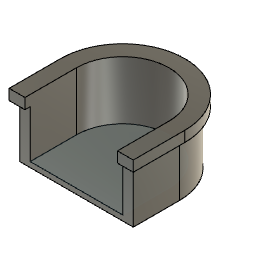
turnknob holder v5 (Autodesk Fusion 360 design; units mm, degrees)
Autodesk Fusion 360 part; units mm, degrees
note: some values were not read from the file. Chosen so that the rebuilt part matches the saved one: which face or edge a step refers to. Set by a fixed rule: which sketch regions a step uses.
sketch "Sketch1" plane through (0, 0, 0) normal (0, 0, 1) x (1, 0, 0)
  line L0 (-8.75, 0) -> (-8.75, -8.75)
  line L1 (-8.75, -8.75) -> (0, -8.75)
  line L2 (0, -8.75) -> (8.75, -8.75)
  line L3 (8.75, -8.75) -> (8.75, 0)
  arc A0 (8.75, 0) -> (-8.75, 0) centre (0, 0) ccw
  line L4 (10.75, -8.75) -> (10.75, 0)
  arc A1 (10.75, 0) -> (-10.75, 0) centre (0, 0) ccw
  line L5 (-10.75, 0) -> (-10.75, -8.75)
  line L6 (-8.75, -8.75) -> (-10.75, -8.75)
  line L7 (8.75, -8.75) -> (10.75, -8.75)
  dimension "d8" = 17.5
  dimension "d9" = 8.75
  dimension "d10" = 8.75
  dimension "d25" = 2
  constraint coincident A0.centre A1.centre
  constraint tangent L0 A0
  constraint tangent L1 A0
  constraint tangent L2 A0
  constraint tangent L3 A0
  constraint perpendicular L5 L6
  constraint perpendicular L4 L7
  constraint parallel L3 L4
  constraint concentric A0 A1
  constraint parallel L0 L5
  constraint tangent A1 L5
  constraint tangent L4 A1
  measures "d8" diameter of A0
  measures "d9" distance of L0.start L0.end
  measures "d10" distance of L1.end L2.end
  measures "d25" distance of L0.end L5.end
extrude "Extrude4" add sketch "Sketch1" along normal blind 1
sketch "Sketch4" plane through (0, 0, 1) normal (0, 0, 1) x (-1, 0, 0)
  line L0 (10.75, 8.75) -> (-10.75, 8.75)
  line L1 (-8.75, 7.75) -> (-8.75, 0)
  arc A0 (-8.75, 0) -> (8.75, 0) centre (0, 0) ccw
  line L2 (8.75, 0) -> (8.75, 7.75)
  line L3 (8.75, 7.75) -> (8.75, 8.75)
  line L4 (-8.75, 7.75) -> (-8.75, 8.75)
  line L5 (-8.75, 8.75) -> (8.75, 8.75)
  line L6 (-10.75, 8.75) -> (-10.75, 0)
  arc A1 (-10.75, 0) -> (10.75, 0) centre (0, 0) ccw
  line L7 (10.75, 0) -> (10.75, 8.75)
  constraint coincident L0 L3.end
  constraint perpendicular L0 L3
  constraint coincident L0 L4.end
  constraint perpendicular L0 L4
  constraint tangent L1 A0
  constraint tangent A0 L2
extrude "Extrude5" add sketch "Sketch4" along normal blind 10.5 contours L0 L1 A0 L2 L3 L4 L6 A1 L7
extrude "Extrude7" add 1 faces at (10.0833, -5.8333, 11.5) along direction (0, 0, 1) blind 0.5
sketch "Sketch7" plane through (0, 0, 12) normal (0, 0, 1) x (-1, 0, 0)
  line L0 (-10.75, 8.75) -> (-10.75, 0)
  arc A0 (-10.75, 0) -> (10.75, 0) centre (0, 0) ccw
  line L1 (10.75, 0) -> (10.75, 8.75)
  line L2 (10.75, 8.75) -> (8.75, 8.75)
  line L3 (8.75, 8.75) -> (8.75, 0)
  arc A1 (-8.75, 0) -> (8.75, 0) centre (0, 0) ccw
  line L4 (-8.75, 0) -> (-8.75, 8.75)
  line L5 (-8.75, 8.75) -> (-10.75, 8.75)
  arc A2 (-11.75, 0) -> (11.75, 0) centre (0, 0) ccw
  line L6 (11.75, 0) -> (11.75, 9.75)
  line L7 (11.75, 9.75) -> (7.75, 9.75)
  line L8 (7.75, 9.75) -> (7.75, 0)
  arc A3 (-7.75, 0) -> (7.75, 0) centre (0, 0) ccw
  line L9 (-7.75, 0) -> (-7.75, 9.75)
  line L10 (-7.75, 9.75) -> (-11.75, 9.75)
  line L11 (-11.75, 9.75) -> (-11.75, 0)
  dimension "d28" = 1
extrude "Extrude8" add sketch "Sketch7" against normal blind 2
sketch "Sketch8" plane through (0, 0, 12) normal (0, 0, 1) x (-1, 0, 0)
  line L0 (-7.75, 0) -> (-7.75, 9.75)
  line L1 (-7.75, 9.75) -> (-11.75, 9.75)
  line L2 (-11.75, 9.75) -> (-11.75, 0)
  arc A0 (-11.75, 0) -> (11.75, 0) centre (0, 0) ccw
  line L3 (11.75, 0) -> (11.75, 9.75)
  line L4 (11.75, 9.75) -> (7.75, 9.75)
  line L5 (7.75, 9.75) -> (7.75, 0)
  arc A1 (-7.75, 0) -> (7.75, 0) centre (0, 0) ccw
  circle A2 centre (0, 0) radius 8.75
  line L6 (8.75, 9.75) -> (7.75, 9.75)
  line L7 (7.75, 9.75) -> (-7.75, 9.75)
  line L8 (-7.75, 9.75) -> (-8.75, 9.75)
  line L9 (-8.75, 9.75) -> (-8.75, 0)
  line L10 (8.75, 9.75) -> (8.75, 0)
  dimension "d31" = 17.5
  dimension "d32" = 1
  constraint concentric A0 A2
  constraint coincident A2 L10.end
  constraint coincident L4 L6.start
  constraint coincident L4.end L5.start
  constraint perpendicular L5 L6
  constraint coincident L0.end L1.start
  constraint coincident L1 L8.end
  constraint coincident A2 L9.end
  constraint tangent A2 L9
  constraint tangent A2 L10
  measures "d31" diameter of A2
  measures "d32" distance of L0.end L8.end
extrude "Extrude9" cut sketch "Sketch8" against normal blind 11 contours L0 L5 A1 A2 | L0 L5 A1 A2 | L0 L1 A2 L8 L9 | L4 L5 A2 L6 L10
sketch "Sketch9" plane through (0, 0, 1) normal (0, 0, 1) x (-1, 0, 0)
  line L0 (8.75, 8.75) -> (-8.75, 8.75)
  line L1 (-8.75, 8.75) -> (-8.75, 0)
  arc A0 (-8.75, 0) -> (8.75, 0) centre (0, 0) ccw
  line L2 (8.75, 0) -> (8.75, 8.75)
sketch "Sketch5" plane through (0, 0, 9.5) normal (0, 0, 1) x (-1, 0, 0)
  line L0 (-8.75, 0) -> (-8.75, 8.75)
  line L1 (-8.75, 8.75) -> (-9.75, 8.75)
  line L2 (-9.75, 8.75) -> (-9.75, 0)
  arc A0 (-9.75, 0) -> (9.75, 0) centre (0, 0) ccw
  line L3 (9.75, 0) -> (9.75, 8.75)
  line L4 (9.75, 8.75) -> (8.75, 8.75)
  line L5 (8.75, 8.75) -> (8.75, 0)
  arc A1 (-8.75, 0) -> (8.75, 0) centre (0, 0) ccw
  arc A2 (-10.75, 0) -> (10.75, 0) centre (0, 0) ccw
  line L6 (-10.75, 0) -> (-10.75, 8.75)
  line L7 (-10.75, 8.75) -> (-9.75, 8.75)
  line L8 (10.75, 0) -> (10.75, 8.75)
  line L9 (10.75, 8.75) -> (9.75, 8.75)
  dimension "d19" = 1
  dimension "d20" = 8.75
  dimension "d21" = 8.75
  constraint parallel L2 L6
  constraint coincident L1.end L2.start
  constraint perpendicular L2 L7
  constraint tangent A2 L8
  constraint vertical L8
  constraint coincident L3.end L4.start
  measures "d20" distance of A2.start L6.end
  measures "d21" distance of A2.end L8.end
extrude "Extrude6" [suppressed]
sketch "Sketch6" plane through (0, 0, 9.5) normal (0, 0, 1) x (-1, 0, 0)
  line L0 (-8.75, 0) -> (-8.75, 8.75)
  line L1 (-8.75, 8.75) -> (-10.75, 8.75)
  line L2 (-10.75, 8.75) -> (-10.75, 0)
  arc A0 (-10.75, 0) -> (10.75, 0) centre (0, 0) ccw
  line L3 (10.75, 0) -> (10.75, 8.75)
  line L4 (10.75, 8.75) -> (8.75, 8.75)
  line L5 (8.75, 8.75) -> (8.75, 0)
  arc A1 (-8.75, 0) -> (8.75, 0) centre (0, 0) ccw
extrude "Extrude1" [suppressed]
sketch "Sketch2" plane through (0, 0, 1) normal (0, 0, 1) x (-1, 0, 0)
  line L0 (8, 8) -> (-8, 8)
  line L1 (-8, 8) -> (-8, 9)
  line L2 (-8, 9) -> (-9, 9)
  line L3 (-9, 9) -> (-9, 0)
  arc A0 (-9, 0) -> (9, 0) centre (0, 0) ccw
  line L4 (9, 0) -> (9, 9)
  line L5 (9, 9) -> (8, 9)
  line L6 (8, 9) -> (8, 8)
  line L7 (8, 0) -> (8, 9)
  line L8 (-8, 8) -> (-8, 9)
  line L9 (-8, 9) -> (-9, 9)
  line L10 (-9, 9) -> (-9, 0)
  line L11 (8, 9) -> (9, 9)
  line L12 (9, 0) -> (9, 9)
  arc A1 (-9, 0) -> (9, 0) centre (0, 0) ccw
  arc A2 (-8, 0) -> (8, 0) centre (0, 0) ccw
  line L13 (-8, 0) -> (-8, 9)
  dimension "d5" = 16
  constraint concentric A0 A2
  constraint coincident L5.end L6.start
  constraint coincident L1.end L2.start
  constraint coincident L2.end L3.start
  constraint coincident L3.end A0.start
  constraint coincident L4.end L5.start
  constraint coincident A0.end L4.start
  constraint concentric A1 A2
  constraint coincident L3.end A1
  measures "d5" diameter of A2
extrude "Extrude2" [suppressed]
sketch "Sketch3" plane through (0, 0, 9) normal (0, 0, 1) x (-1, 0, 0)
  arc A0 (-8, 0) -> (8, 0) centre (0, 0) ccw
  line L0 (-8, 0) -> (-8, 9)
  line L1 (-8, 9) -> (-9, 9)
  line L2 (-9, 9) -> (-9, 0)
  arc A1 (-9, 0) -> (9, 0) centre (0, 0) ccw
  line L3 (9, 0) -> (9, 9)
  line L4 (9, 9) -> (8, 9)
  line L5 (8, 9) -> (8, 0)
  line L6 (8, 8) -> (9, 8)
  line L7 (9, 8) -> (9, 9)
  line L8 (9, 9) -> (8, 9)
  line L9 (8, 8) -> (8, 9)
  line L10 (-8, 8) -> (-8, 9)
  line L11 (-8, 9) -> (-9, 9)
  line L12 (-9, 9) -> (-9, 8)
  line L13 (-9, 8) -> (-8, 8)
  constraint coincident L5 L6.start
  constraint coincident L3 L6.end
  constraint perpendicular L3 L6
  constraint coincident L3.end L4.start
  constraint coincident L4.end L5.start
  constraint coincident L0 L10.start
  constraint coincident L0.end L1.start
  constraint coincident L1.end L2.start
  constraint coincident L2 L12.end
  constraint parallel L2 L12
extrude "Extrude3" [suppressed]
